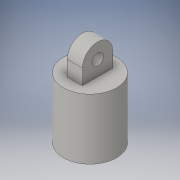
# Autodesk Inventor part: shock absorber top
Saved by Autodesk Inventor 2016 (Build 200138000, 138)
## iProperties
Created: 2017-06-27
Part Number: shock absorber top
Material: Generic
Document SubType Name: Modeling
Designer: andon
Density: 1 g/cm^3
Appearance: Default
Author: andon
Autodesk Inventor part; units mm, degrees
ref_plane "YZ Plane" through (0, 0, 0) normal (1, 0, 0) x (0, 1, 0)
ref_plane "XZ Plane" through (0, 0, 0) normal (0, 1, 0) x (-1, 0, 0)
ref_plane "XY Plane" through (0, 0, 0) normal (0, 0, 1) x (1, 0, 0)
sketch "Sketch1" plane through (0, 0, 0) normal (1, 0, 0) x (0, 1, 0)
  line L0 (-50.8, 44.45) -> (50.8, 44.45)
  line L1 (50.8, 44.45) -> (50.8, 41.275)
  line L2 (-50.8, 41.275) -> (-50.8, 44.45)
  line L3 (-50.8, 44.45) -> (-47.1714, 41.275) construction
  line L4 (50.8, 41.275) -> (-50.8, 41.275)
  line L5 (50.8, 44.45) -> (47.1714, 41.275) construction
  line L6 (-71.12, 0) -> (71.12, 0) projected
  point P0 (0, 0)
  constraints: 12 end point, 3 point on line, 2 horizontal, 1 parallel, 1 perpendicular
revolve "Revolution1" add sketch "Sketch1" angle 360 about axis through (0, -10, 0) along (0, 1, 0)
sketch "Sketch2" plane through (0, 50.8, 0) normal (0, 1, 0) x (1, 0, 0)
  circle A0 centre (0, 0) radius 44.45
  constraints: 1 centre point, 1 coincident
extrude "Extrusion1" add sketch "Sketch2" against normal blind 6.35
sketch "Sketch3" plane through (0, -50.8, 0) normal (0, -1, 0) x (1, 0, 0)
  circle A0 centre (0, 0) radius 44.45
  constraints: 1 centre point, 1 coincident
extrude "Extrusion2" add sketch "Sketch3" against normal blind 6.35
sketch "Sketch4" plane through (0, -50.8, 0) normal (0, -1, 0) x (1, 0, 0)
  circle A0 centre (0, 0) radius 44.45 projected
  circle A1 centre (0, 0) radius 19.05
  constraints: 1 centre point, 1 coincident
extrude "Extrusion3" cut sketch "Sketch4" against normal blind 12.7 contours A1
sketch "Sketch5" plane through (0, 50.8, 0) normal (0, 1, 0) x (1, 0, 0)
  line L0 (-25.4, 25.4) -> (25.4, 25.4)
  line L1 (25.4, 25.4) -> (25.4, -25.4)
  line L2 (25.4, -25.4) -> (-25.4, -25.4)
  line L3 (-25.4, -25.4) -> (-25.4, 25.4)
  line L4 (-25.4, 25.4) -> (25.4, -25.4) construction
  line L5 (25.4, 25.4) -> (-25.4, -25.4) construction
  line L6 (-12.7, 25.4) -> (12.7, 25.4)
  line L7 (12.7, 25.4) -> (12.7, -25.4)
  line L8 (12.7, -25.4) -> (-12.7, -25.4)
  line L9 (-12.7, -25.4) -> (-12.7, 25.4)
  line L10 (-12.7, 25.4) -> (12.7, -25.4) construction
  line L11 (12.7, 25.4) -> (-12.7, -25.4) construction
  point P0 (0, 0)
  dimension "d9" = 50.8
  dimension "d10" = 50.8
  constraints: 24 end point, 4 midpoint, 4 parallel, 2 horizontal, 2 perpendicular, 1 point on line
  measures "d9" distance of L1.end L2.end
  measures "d10" distance of L0.end L1.end
extrude "Extrusion6" add sketch "Sketch5" along normal blind 50.8 contours L0 L7 L2 L9
fillet "Fillet2" radius 25.4 2 edges at (0, 101.6, 25.4) (0, 101.6, -25.4)
sketch "Sketch7" plane through (12.7, 50.8, 25.4) normal (1, 0, 0) x (0, 0, -1)
  arc A0 (50.8, 25.4) -> (0, 25.4) centre (25.4, 25.4) ccw projected
  circle A1 centre (25.4, 25.4) radius 9.525
  point P0 (25.4, -50.8)
  dimension "d20" = 19.05
  constraints: 1 centre point, 1 coincident
  measures "d20" diameter of A1
extrude "Extrusion7" cut sketch "Sketch7" against normal blind 50.8
body "Solid1"
